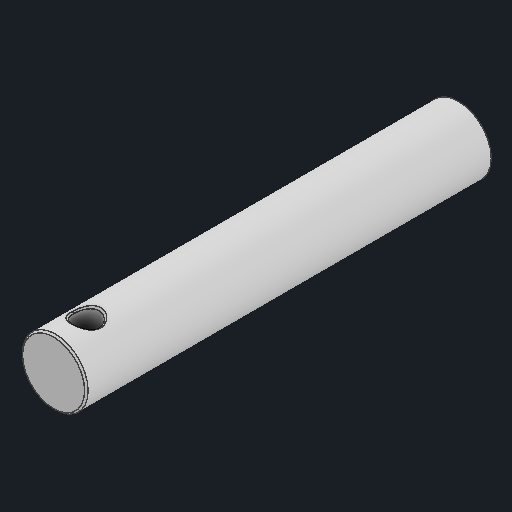
# Autodesk Inventor part: FA-RMS-15-12-4-Piston
Saved by Autodesk Inventor 2025.2 (Build 292293000, 293)
## iProperties
Created: 2025-09-26
Part Number: FA-RMS-15-12-4-Piston
Material: Generic
Document SubType Name: Modeling
Designer: valer
Density: 1 g/cm^3
Appearance: Default
Author: valer
Autodesk Inventor part; units mm, degrees
ref_plane "YZ Plane" through (0, 0, 0) normal (1, 0, 0) x (0, 1, 0)
ref_plane "XY Plane" through (0, 0, 0) normal (0, 0, 1) x (1, 0, 0)
sketch "Base" plane through (0, 0, 0) normal (0, 0, 1) x (1, 0, 0)
  circle A0 centre (0, 0) radius 9.525
  dimension "d0" = 19.05
  constraints: 1 centre point, 1 coincident
  measures "d0" diameter of A0
extrude "BaseFeature" add sketch "Base" along normal blind 117.475
chamfer "BaseChamferFeature" distance 0.508 angle 45 1 edges at (-9.525, 0, 117.475)
sketch "MountHole" plane through (0, 0, 0) normal (0, 1, 0) x (-1, 0, 0)
  line L0 (-9.017, 117.475) -> (9.017, 117.475) construction
  line L1 (0, 117.475) -> (0, 111.633) construction
  line L2 (0, 111.633) -> (0, 107.95) construction
  circle A0 centre (0, 107.95) radius 3.683
  point P0 (0, 0)
  dimension "d6" = 5.842
  dimension "d7" = 3.683
  constraints: 4 end point, 2 vertical, 1 coincident, 1 midpoint, 1 vertical alignment, 2 other
  measures "d6" distance of L1.start L1.end
  measures "d7" distance of L1.end L2.end
extrude "MountHoleFeature" cut sketch "MountHole" along normal through all both and the other way through all
chamfer "MountHoleChamferFeature" distance 0.507 angle 45 2 edges at (3.683, -8.7841, 107.9534) (3.683, 8.7841, 107.9534)
ref_plane "MountPlane" through (0, -10, 0) normal (0, -1, 0) x (1, 0, 0)
body "Solid1"
